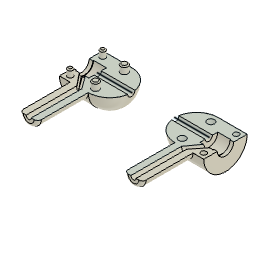
OpenEarable ExG Earplugs (Autodesk Fusion 360 design; units mm, degrees)
Autodesk Fusion 360 part; units mm, degrees
note: some values were not read from the file. Chosen so that the rebuilt part matches the saved one: which face or edge a step refers to; that a step has no effect; which pieces of a blend or face edit are solid. Set by a fixed rule: which sketch regions a step uses.
sketch "Sketch1" plane through (0, 0, 0) normal (0, 0, 1) x (1, 0, 0)
  line L0 (-4, 6) -> (4, 6)
  line L1 (4, 6) -> (4, -6)
  line L2 (4, -6) -> (-4, -6)
  line L3 (-4, -6) -> (-4, 6)
  line L4 (1.75, 0) -> (22.5, 0)
  line L5 (0, 1.75) -> (0, 22.5)
  line L6 (4, 6) -> (4, -6)
  arc A0 (4, -6) -> (4, 6) centre (4, 0) ccw
  line L7 (-4, 6) -> (-10, 6)
  line L8 (-14, 2) -> (-14, -2.0005)
  line L9 (-10, -6) -> (-4, -6)
  line L10 (-4, -6) -> (-4, 6)
  line L11 (-4, 1) -> (-14, 1)
  line L12 (-4, -1) -> (-14, -1)
  line L13 (-10, 6) -> (-10, -6)
  arc A1 (-10, 6) -> (-14, 2) centre (-10, 2) ccw
  arc A2 (-14, -1.9995) -> (-10, -6) centre (-10, -2) ccw
  line L14 (-1, -6) -> (4, -6)
  line L15 (4, -6) -> (4, -20)
  line L16 (4, -20) -> (-1, -20)
  line L17 (-1, -20) -> (-1, -6)
  line L18 (0.8, -20) -> (0.8, -6)
  line L19 (2.2, -20) -> (2.2, -6)
  line L20 (-4, 2.45) -> (0.6, 2.45)
  line L21 (0.6, 2.45) -> (0.6, -2.45)
  line L22 (0.6, -2.45) -> (-4, -2.45)
  line L23 (-4, -2.45) -> (-4, 2.45)
  line L24 (-4, 2.25) -> (-3, 2.25)
  line L25 (-3, 2.25) -> (-3, -2.25)
  line L26 (-3, -2.25) -> (-4, -2.25)
  line L27 (-4, -2.25) -> (-4, 2.25)
  line L28 (0.8, -6) -> (-2.025, -2.45)
  line L29 (2.2, -6) -> (-0.375, -2.45)
  line L30 (-2.9984, -2.45) -> (-2.9984, 2.45)
  circle A3 centre (4, -4) radius 1
  circle A4 centre (4, 4) radius 1
  circle A5 centre (-2.5, 4.5) radius 0.75
  circle A6 centre (-2.5, -4.5) radius 0.75
  dimension "d1" = 8
  dimension "d2" = 12
  dimension "d3" = 5
  dimension "d4" = 5
  dimension "d5" = 4
  dimension "d6" = 14
  dimension "d7" = 5
  dimension "d10" = 1.8
  dimension "d11" = 1.8
  dimension "d12" = 4.9
  dimension "d13" = 4.6
  dimension "d14" = 3.6
  dimension "d15" = 4.5
  dimension "d16" = 0.975
  dimension "d18" = 1.65
  dimension "d19" = 2
  dimension "d20" = 2
  dimension "d21" = 1.5
  dimension "d22" = 1.5
  dimension "d23" = 2
  dimension "d24" = 2
  dimension "d25" = 1.5
  dimension "d26" = 1.5
  dimension "d27" = 1.5
  dimension "d28" = 1.5
  constraint horizontal L0
  constraint vertical L1
  constraint horizontal L2
  constraint vertical L3
  constraint symmetric L0 L2 L4
  constraint symmetric L1 L3 L5
  constraint tangent L0 A0
  constraint horizontal L7
  constraint vertical L8
  constraint horizontal L9
  constraint vertical L10
  constraint coincident L3 L11.start
  constraint coincident L8 L11.end
  constraint perpendicular L8 L11
  constraint coincident L10 L12.start
  constraint coincident L8 L12.end
  constraint perpendicular L8 L12
  constraint perpendicular L9 L13
  constraint coincident A2 L8.end
  constraint horizontal L14
  constraint vertical L15
  constraint horizontal L16
  constraint vertical L17
  constraint coincident L2 L14.start
  constraint coincident L16 L18.start
  constraint coincident L14 L18.end
  constraint perpendicular L14 L18
  constraint coincident L16 L19.start
  constraint coincident L2 L19.end
  constraint perpendicular L2 L19
  constraint coincident L8 A2.start
  constraint horizontal L20
  constraint vertical L21
  constraint horizontal L22
  constraint vertical L23
  constraint coincident L3 L20.start
  constraint symmetric L4 L20 L22
  constraint horizontal L24
  constraint vertical L25
  constraint horizontal L26
  constraint vertical L27
  constraint coincident L23 L24.start
  constraint symmetric L4 L24 L26
  constraint coincident L22 L28.end
  constraint coincident L22 L29.end
  constraint coincident L22 L30.start
  constraint coincident L20 L30.end
  constraint perpendicular L20 L30
  constraint coincident L1 A3.centre
  constraint coincident L1 A4.centre
  measures "d1" distance of L0.start L0.end
  measures "d2" distance of L0.end L1.end
  measures "d3" distance of L7 L11
  measures "d4" distance of L9 L12
  measures "d5" distance of L8 L13
  measures "d6" distance of L1.end L15.end
  measures "d7" distance of L15.end L16.end
  measures "d10" distance of L15 L19
  measures "d11" distance of L17 L18
  measures "d12" distance of L20.end L21.end
  measures "d13" distance of L20.start L20.end
  measures "d14" distance of L21 L25
  measures "d15" distance of L24.end L25.end
  measures "d16" distance of L21.end L29.end
  measures "d18" distance of L28.end L29.end
  measures "d19" diameter of A3
  measures "d20" diameter of A4
  measures "d21" diameter of A5
  measures "d22" diameter of A6
  measures "d23" distance of L0.end A4.centre
  measures "d24" distance of L1.end A3.centre
  measures "d25" distance of L2 A6.centre
  measures "d26" distance of L10 A6.centre
  measures "d27" distance of L0 A5.centre
  measures "d28" distance of L10 A5.centre
extrude "Extrude1" add sketch "Sketch1" along normal blind 5.35 contours L2 L14 L16 L18 L19 | L2 L14 L22 L28 L29 makes body 1
extrude "Extrude2" add sketch "Sketch1" along normal blind 6 contours L0 L3 L5 L10 L20 | L0 L1 L2 L5 L6 L14 L20 L21 L22 L29 A3 A4 | L1 L4 L6 A0 A4 | L1 L4 L6 A0 A3 | L2 L14 L15 L16 L19 | L2 L3 L10 L14 L22 L28 | L2 L14 L16 L17 L18 bodies 1
extrude "Extrude3" cut sketch "Sketch1" along normal blind 3.5 contours L2 L14 L15 L16 L19 | L2 L14 L16 L18 L19 | L2 L14 L16 L17 L18 bodies 1
extrude "Extrude4" add sketch "Sketch1" along normal blind 3.55 contours L20 L21 L22 L25 L30 bodies 1
extrude "Extrude5" add sketch "Sketch1" along normal blind 3.75 separate body contours L3 L10 L23 L24 L25 L26 L27 L30 makes body 2
extrude "Extrude6" add sketch "Sketch1" along normal blind 3.55 contours L3 L10 L20 L23 L24 L30 | L3 L10 L23 L24 L25 L26 L27 L30 | L3 L10 L22 L23 L26 L30 bodies 1 2
fillet "Fillet1" radius 2.5 1 edges at (4, -13, 3.5) on bodies 1
fillet "Fillet2" radius 2.5 1 edges at (-1, -13, 3.5) on bodies 1
fillet "Fillet3" radius 0.2 1 edges at (0.8, -13, 5.35) on bodies 1
fillet "Fillet4" radius 0.2 1 edges at (2.2, -13, 5.35) on bodies 1
fillet "Fillet5" [no effect]
fillet "Fillet6" radius 0.5 1 edges at (-0.5125, -4.3507, 5.35) on bodies 1
sketch "Sketch2" plane through (0, 0, 3.55) normal (0, 0, 1) x (-1, 0, 0)
  line L0 (4, 2.45) -> (-0.6, 2.45)
  line L1 (-0.6, 2.45) -> (-0.6, -2.45)
  line L2 (-0.6, -2.45) -> (4, -2.45)
  line L3 (4, -2.45) -> (4, -2.25)
  line L4 (4, -2.25) -> (3, -2.25)
  line L5 (3, -2.25) -> (3, 2.25)
  line L6 (3, 2.25) -> (4, 2.25)
  line L7 (4, 2.25) -> (4, 2.45)
  line L8 (3, -2.45) -> (3, 2.45)
  constraint coincident L2 L8.start
  constraint coincident L0 L8.end
  constraint perpendicular L0 L8
extrude "Extrude7" add sketch "Sketch2" along normal blind 2.45 contours L2 L3 L4 L8 bodies 1
extrude "Extrude8" add sketch "Sketch2" along normal blind 2.45 contours L0 L6 L7 L8 bodies 1
fillet "Fillet7" radius 2.25 1 edges at (-3.5, 2.25, 3.75) on bodies 1
fillet "Fillet8" radius 2.25 1 edges at (-3.5, -2.25, 3.75) on bodies 1
fillet "Fillet9" radius 2.45 1 edges at (-1.2, 2.45, 3.55) on bodies 1
fillet "Fillet10" radius 2.45 1 edges at (-1.2, -2.45, 3.55) on bodies 1
extrude "Extrude9" add sketch "Sketch1" along normal blind 10 contours L1 L6 A4 | L1 L6 A4 | L1 L6 A3 | L1 L6 A3 | A5 | A6 bodies 1
fillet "Fillet11" radius 5.99 3 edges at (0, 6, 0) (10, 0, 0) (0, -6, 0) on bodies 1
extrude "Extrude10" cut 4 faces at (-2.3537, 4.6756, 10) (4.2444, 4.2267, 10) (-2.532, -4.6947, 10) (3.8663, -4.4333, 10) along direction (0, 0, -1) blind 2 on bodies 1 bodies 1
fillet "Fillet12" radius 0.3 4 edges at (-3.1992, 4.7712, 8) (3.0677, 4.3616, 8) (-3.1992, -4.2288, 8) (3.0677, -3.6384, 8) on bodies 1
fillet "Fillet13" radius 1 1 edges at (1.5, -20, 3.5) on bodies 1
ref_plane "WorkPlane1" through (16, 0, 3) normal (-1, 0, 0) x (0, -1, 0)
mirror "Mirror1" about plane through (16, 0, 3) normal (-1, 0, 0) of bodies 1 makes body 3
delete_face "DeleteFace3" 1 faces at (28.9359, 4.3124, 7.7884) on bodies 3
delete_face "DeleteFace4" 1 faces at (34.8397, 5.1626, 7.7568) on bodies 3
delete_face "DeleteFace5" 1 faces at (34.8397, -3.8374, 7.7568) on bodies 3
delete_face "DeleteFace6" 1 faces at (28.9359, -3.6876, 7.7884) on bodies 3
extrude "Extrude17" cut 4 faces at (28.2638, -4.1785, 8) (27.7246, 3.8122, 8) (34.7226, 4.4746, 8) (34.6196, -4.049, 8) along direction (0, 0, -1) blind 4 on bodies 3 bodies 3
delete_face "DeleteFace7" 1 faces at (2.0401, -10.5171, 5.3541) on bodies 1
delete_face "DeleteFace8" 1 faces at (0.9768, -10.8171, 5.3513) on bodies 1
delete_face "DeleteFace9" 1 faces at (0.0123, -4.3127, 5.3543) on bodies 1
extrude "Extrude18" cut 1 faces at (1.2667, -10.6667, 5.35) along direction (0, 0, -1) blind 0.05 on bodies 1 bodies 1
fillet "Fillet15" radius 0.7 1 edges at (0.8, -13, 5.3) on bodies 1
fillet "Fillet16" radius 0.7 2 edges at (0.8807, -4.1811, 5.3) (2.2, -13, 5.3) on bodies 1
fillet "Fillet17" radius 0.4 1 edges at (-0.2974, -4.6209, 5.3) on bodies 1
delete_face "DeleteFace10" 1 faces at (31.1986, -15.334, 5.5264) on bodies 3
delete_face "DeleteFace11" 1 faces at (29.9748, -10.5043, 5.3516) on bodies 3
delete_face "DeleteFace12" 1 faces at (32.7396, -3.3491, 5.3529) on bodies 3
extrude "Extrude19" cut 1 faces at (30.7333, -10.6667, 5.35) along direction (0, 0, -1) blind 0.05 on bodies 3 bodies 3
fillet "Fillet18" radius 0.7 2 edges at (29.8, -13, 5.3) (31.1193, -4.1811, 5.3) on bodies 3
fillet "Fillet19" radius 0.7 1 edges at (31.2, -13, 5.3) on bodies 3
fillet "Fillet20" radius 0.4 1 edges at (32.2974, -4.6209, 5.3) on bodies 3
sketch "Sketch3" plane through (0, 0, 6) normal (0, 0, 1) x (-1, 0, 0)
  arc A0 (-3, 20) -> (-4, 19) centre (-3, 19) ccw
  line L0 (-4, 19) -> (-4, 6)
  arc A1 (-4, 6) -> (-4, -6) centre (-4, 0) ccw
  line L1 (-4, -6) -> (4, -6)
  line L2 (4, -6) -> (4, -2.25)
  line L3 (4, -2.25) -> (3, -2.25)
  line L4 (3, -2.25) -> (3, -2.45)
  line L5 (3, -2.45) -> (-0.6, -2.45)
  line L6 (-0.6, -2.45) -> (-0.6, 2.45)
  line L7 (-0.6, 2.45) -> (0.375, 2.45)
  line L8 (0.375, 2.45) -> (-2.2, 6)
  line L9 (-2.2, 6) -> (-2.2, 20)
  line L10 (-2.2, 20) -> (-3, 20)
  circle A2 centre (2.5, -4.5) radius 0.75
  circle A3 centre (-4, 4) radius 1
  circle A4 centre (-4, -4) radius 1
  line L11 (-10, 0) -> (-0.6, 0)
  constraint midpoint A1 L11.start
  constraint midpoint L6 L11.end
hole "Hole1" at (0.6, 0, 6) direction (1, 0, 0) diameter 2 depth 11 tip angle 118 bodies 1
sketch "Sketch4" plane through (0, 0, 6) normal (0, 0, 1) x (-1, 0, 0)
  arc A0 (-28, 19) -> (-29, 20) centre (-29, 19) ccw
  line L0 (-29, 20) -> (-29.8, 20)
  line L1 (-29.8, 20) -> (-29.8, 6)
  line L2 (-29.8, 6) -> (-32.375, 2.45)
  line L3 (-32.375, 2.45) -> (-31.4, 2.45)
  line L4 (-31.4, 2.45) -> (-31.4, -2.45)
  line L5 (-31.4, -2.45) -> (-35, -2.45)
  line L6 (-35, -2.45) -> (-35, -2.25)
  line L7 (-35, -2.25) -> (-36, -2.25)
  line L8 (-36, -2.25) -> (-36, -6)
  line L9 (-36, -6) -> (-28, -6)
  arc A1 (-28, -6) -> (-28, 6) centre (-28, 0) ccw
  line L10 (-28, 6) -> (-28, 19)
  circle A2 centre (-34.5, -4.5) radius 0.75
  circle A3 centre (-28, 4) radius 1
  circle A4 centre (-28, -4) radius 1
  line L11 (-22, 0) -> (-31.4, 0)
  constraint midpoint A1 L11.start
  constraint midpoint L4 L11.end
hole "Hole2" at (31.4, 0, 6) direction (-1, 0, 0) diameter 2 depth 12.5 tip angle 118 bodies 3
named bodies: "left earpiece", "right earpiece"
